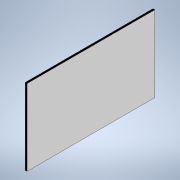
# Autodesk Inventor part: ekran
Saved by Autodesk Inventor 2020 (Build 240168000, 168)
## iProperties
Created: 2019-11-30
Part Number: ekran
Material: Ogólny
Document SubType Name: Modeling
Designer: hubslo
Density: 1 g/cm^3
Appearance: Domyślna
Author: hubslo
Autodesk Inventor part; units mm, degrees
ref_plane "YZ Plane" through (0, 0, 0) normal (1, 0, 0) x (0, 1, 0)
ref_plane "XZ Plane" through (0, 0, 0) normal (0, 1, 0) x (-1, 0, 0)
ref_plane "XY Plane" through (0, 0, 0) normal (0, 0, 1) x (1, 0, 0)
sketch "Szkic1" plane through (0, 0, 0) normal (1, 0, 0) x (0, 1, 0)
  line L0 (-49, 82.5) -> (49, 82.5)
  line L1 (49, 82.5) -> (49, -82.5)
  line L2 (49, -82.5) -> (-49, -82.5)
  line L3 (-49, -82.5) -> (-49, 82.5)
  line L4 (-49, 82.5) -> (49, -82.5) construction
  line L5 (49, 82.5) -> (-49, -82.5) construction
  point P0 (0, 0)
  dimension "d0" = 98
  dimension "d1" = 165
  constraints: 12 end point, 2 midpoint, 2 parallel, 1 horizontal, 1 perpendicular
  measures "d0" distance of L1.end L2.end
  measures "d1" distance of L0.end L1.end
extrude "Wyciągnięcie proste1" add sketch "Szkic1" along normal blind 2.6
